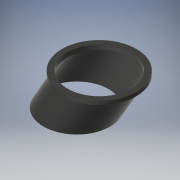
# Autodesk Inventor part: Water Bottle Ring
Saved by Autodesk Inventor 2019 (Build 230136000, 136)
## iProperties
Created: 2020-12-25
Part Number: Water Bottle Ring
Material: Acetal Resin, Black
Document SubType Name: Modeling
Designer: John
Density: 1.425 g/cm^3
Appearance: Smooth - Black
Author: John
Autodesk Inventor part; units mm, degrees
ref_plane "YZ Plane" through (0, 0, 0) normal (1, 0, 0) x (0, 1, 0)
ref_plane "XZ Plane" through (0, 0, 0) normal (0, 1, 0) x (-1, 0, 0)
ref_plane "XY Plane" through (0, 0, 0) normal (0, 0, 1) x (1, 0, 0)
sketch "Sketch1" plane through (0, 0, 0) normal (0, 1, 0) x (-1, 0, 0)
  circle A0 centre (0, 0) radius 57.15 construction
  circle A1 centre (0, 0) radius 63.5
  circle A2 centre (0, 0) radius 56.896
  circle A3 centre (0, 0) radius 50.8 construction
  circle A4 centre (0, 0) radius 53.975
  dimension "d0" = 114.3
  dimension "d1" = 127
  dimension "d2" = 113.792
  dimension "d3" = 101.6
  dimension "d4" = 107.95
  constraints: 5 centre point, 5 coincident
  measures "d0" diameter of A0
  measures "d1" diameter of A1
  measures "d2" diameter of A2
  measures "d3" diameter of A3
  measures "d4" diameter of A4
extrude "Extrusion1" add sketch "Sketch1" along normal blind 6.35 contours A1 | A2
extrude "Extrusion2" add sketch "Sketch1" against normal blind 1.27 contours A2
sketch "Sketch2" plane through (0, 0, 0) normal (0, 0, 1) x (1, 0, 0)
  line L0 (-56.896, -1.27) -> (56.896, -1.27) projected
  line L1 (-56.896, -1.27) -> (-94.996, -67.2611)
  line L2 (-56.896, -1.27) -> (19.304, -1.27) construction
  point P0 (0, 0)
  dimension "d9" = 120
  dimension "d10" = 76.2
  constraints: 4 end point, 1 equal length, 1 horizontal
  measures "d9" angle of L1 L2
  measures "d10" distance of L0.start L1.end
ref_plane "Work Plane1" through (-94.996, -67.2611, 0) normal (0, -1, 0) x (1, 0, 0)
sketch "Sketch3" plane through (-94.996, -67.2611, 0) normal (0, -1, 0) x (1, 0, 0)
  circle A0 centre (56.896, 0) radius 56.896
  line L0 (38.1, 0) -> (0, 0) projected
  line L1 (0, 0) -> (0, -9.2557)
  circle A1 centre (56.896, 0) radius 53.975
  point P0 (94.996, 0)
  dimension "d11" = 113.792
  dimension "d12" = 107.95
  constraints: 2 centre point, 2 end point, 1 coincident, 1 tangent, 1 vertical
  measures "d11" diameter of A0
  measures "d12" diameter of A1
sketch "Sketch4" plane through (0, -1.27, 0) normal (0, -1, 0) x (1, 0, 0)
  circle A0 centre (0, 0) radius 53.975 projected
  circle A1 centre (0, 0) radius 56.896 projected
loft "Loft1" add profiles "Sketch3", "Sketch4" contours A0 | A1 / A0 | A1
loft "Loft2" cut profiles "Sketch3" section 1 edges at (53.975, -1.27, 0) contours A1
body "Solid1"
